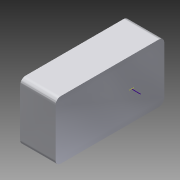
# Autodesk Inventor part: am-2679 671 Mecanum Gearbox
Saved by Autodesk Inventor 2015 (Build 190159000, 159)
## iProperties
Created: 2016-01-21
Part Number: am-2679 671 Mecanum Gearbox
Material: Generic
Document SubType Name: Modeling
Designer: sethbattis
Density: 1 g/cm^3
Appearance: Default
Author: sethbattis
Autodesk Inventor part; units mm, degrees
ref_plane "YZ Plane" through (0, 0, 0) normal (1, 0, 0) x (0, 1, 0)
ref_plane "XZ Plane" through (0, 0, 0) normal (0, 1, 0) x (-1, 0, 0)
ref_plane "XY Plane" through (0, 0, 0) normal (0, 0, 1) x (1, 0, 0)
sketch "Sketch1" plane through (0, 0, 0) normal (1, 0, 0) x (0, 1, 0)
  line L0 (34.1313, 63.5) -> (-34.1313, 63.5)
  line L1 (-34.1313, 63.5) -> (-34.1312, -63.5)
  line L2 (-34.1312, -63.5) -> (34.1313, -63.5)
  line L3 (34.1313, -63.5) -> (34.1313, 63.5)
  line L4 (-47.7838, 0) -> (47.7838, 0) construction
  line L5 (0, -88.9) -> (0, 88.9) construction
  point P0 (0, 0)
  dimension "d0" = 127
  dimension "d1" = 68.2625
  constraints: 8 end point, 2 parallel, 1 horizontal, 1 perpendicular, 2 other
  measures "d0" distance of L2.end L0.start
  measures "d1" distance of L1.end L2.end
extrude "Extrusion1" add sketch "Sketch1" along normal blind 41.275
fillet "Fillet1" radius 6.35 4 edges at (20.6375, 34.1313, 63.5) (20.6375, 34.1313, -63.5) (20.6375, -34.1313, 63.5) (20.6375, -34.1312, -63.5)
sketch "Motor Attachment" plane through (41.275, 0, 0) normal (1, 0, 0) x (0, 0, -1)
  line L0 (63.5, -27.7812) -> (63.5, 27.7813) construction
  line L1 (57.15, 34.1313) -> (-57.15, 34.1313) construction
  line L2 (-57.15, -34.1313) -> (57.15, -34.1312) construction
  line L3 (63.5, -27.7812) -> (63.5, 27.7813) construction
  line L4 (63.5, 0) -> (-63.5, 0) construction
  line L5 (-63.5, 27.7813) -> (-63.5, -27.7813) construction
  line L6 (57.15, 34.1313) -> (-57.15, 34.1313) construction
  line L7 (25.4, 34.1313) -> (25.4, -34.1312) construction
  point P0 (0, 0)
  point P1 (25.4, 0)
  dimension "d5" = 38.1
  constraints: 4 end point, 3 midpoint, 2 point on line, 1 perpendicular
  measures "d5" distance between parallel lines of L0 L7
sketch "Axle Attachment" plane through (0, 0, 0) normal (-1, 0, 0) x (0, 0, 1)
  line L0 (-57.15, 34.1313) -> (57.15, 34.1313) construction
  line L1 (57.15, -34.1313) -> (-57.15, -34.1312) construction
  line L2 (63.5, 27.7813) -> (63.5, -27.7813) construction
  line L3 (-63.5, -27.7812) -> (-63.5, 27.7813) projected
  line L4 (-63.5, 0) -> (63.5, 0) construction
  line L5 (33.3375, 34.1313) -> (33.3375, -34.1313) construction
  point P0 (0, 0)
  point P1 (33.3375, 0)
  dimension "d6" = 30.1625
  constraints: 4 end point, 3 midpoint, 2 point on line, 1 perpendicular
  measures "d6" distance between parallel lines of L2 L5
ref_plane "Work Plane1" through (0, 0, 33.3375) normal (0, -1, 0) x (1, 0, 0)
sketch "Axle Axis" plane through (0, 0, 33.3375) normal (0, -1, 0) x (1, 0, 0)
  line L0 (0, 0) -> (-15.5629, 0)
  point P0 (0, -33.3375)
  constraints: 2 end point, 1 horizontal
ref_plane "Work Plane2" through (41.275, 0, -25.4) normal (0, -1, 0) x (1, 0, 0)
sketch "Motor Axis" plane through (41.275, 0, -25.4) normal (0, -1, 0) x (1, 0, 0)
  line L0 (0, 0) -> (10.3767, 0)
  point P0 (-41.275, 25.4)
  constraints: 2 end point, 1 horizontal
body "Solid1"
